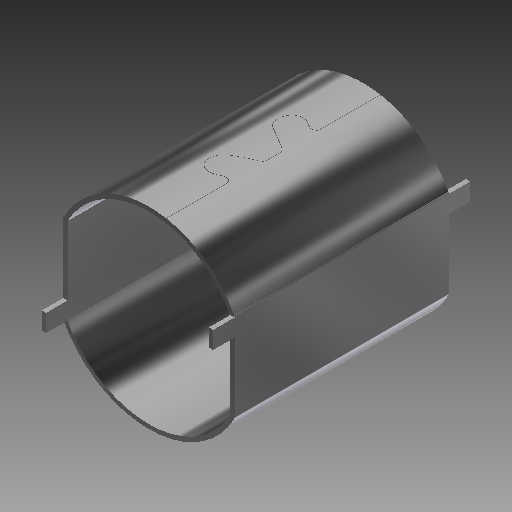
# Autodesk Inventor part: M-001
Saved by Autodesk Inventor 2019 (Build 230136000, 136)
## iProperties
Company: Autodesk Inc.
Created: 2007-10-30
Part Number: M-001
Document SubType Name: Sheet Metal
Designer: Autodesk Inc.
Density: 8 g/cm^3
Mass: 55.2333 g
Surface Area: 142.635 cm^2
Volume: 6.90416 cm^3
Material: Stainless Steel
Description: MOTOR SLEEVE
Sheet Metal Rule: Default
Appearance: Semi-Polished
Component Category: Electrical
Author: Inventor
Autodesk Inventor part; units mm, degrees
ref_plane "YZ Plane" through (0, 0, 0) normal (1, 0, 0) x (0, 1, 0)
ref_plane "XY Plane" through (0, 0, 0) normal (0, 0, 1) x (1, 0, 0)
sketch "Sketch1" plane through (0, 0, 0) normal (0, 0, 1) x (1, 0, 0)
  line L0 (-20, 10.0611) -> (-20, -10.0611)
  line L1 (20, 10.0611) -> (20, -10.0611)
  arc A0 (-19.8831, -10.5315) -> (19.8831, -10.5315) centre (0, 0) ccw
  arc A1 (19.8831, 10.5315) -> (-19.8831, 10.5315) centre (0, 0) ccw
  line L2 (-19, 10.0611) -> (-19, -10.0611)
  arc A2 (-18.9994, -10.0634) -> (19, -10.0623) centre (0, 0) ccw
  line L3 (19, -10.0623) -> (19, 10.0611)
  arc A3 (18.9994, 10.0634) -> (-18.9994, 10.0634) centre (0, 0) ccw
  arc A4 (-18.9994, 10.0634) -> (-19, 10.0611) centre (-18.995, 10.0611) ccw
  arc A5 (19, 10.0611) -> (18.9994, 10.0634) centre (18.995, 10.0611) ccw
  arc A6 (-19, -10.0611) -> (-18.9994, -10.0634) centre (-18.995, -10.0611) ccw
  arc A7 (-19.8831, 10.5315) -> (-20, 10.0611) centre (-18.995, 10.0611) ccw
  arc A8 (-20, -10.0611) -> (-19.8831, -10.5315) centre (-18.995, -10.0611) ccw
  arc A9 (19.8831, -10.5315) -> (20, -10.0611) centre (18.995, -10.0611) ccw
  arc A10 (20, 10.0611) -> (19.8831, 10.5315) centre (18.995, 10.0611) ccw
  dimension "d1" = 40
  dimension "d2" = 20
  dimension "d3" = 22.5
  dimension "d4" = 1
  dimension "d17" = 0.005
  dimension "d19" = 1.005
  dimension "d22" = 22.5
  constraints: 22 point on circle, 14 tangent, 11 centre point, 8 end point, 5 equal radius, 2 parallel, 1 coincident, 1 vertical, 3 other
  measures "d1" distance between parallel lines of L1 L0
  measures "d2" distance from line of L1 point (0, 0)
  measures "d3" radius of A1
  measures "d4" distance between parallel lines of L0 L2
  measures "d17" radius of A4
  measures "d19" radius of A7
  measures "d22" radius of A0
extrude "Extrusion1" add sketch "Sketch1" along normal mid plane 50
ref_plane "Work Plane1" through (0, 22.5, 0) normal (0, 1, 0) x (-1, 0, 0)
sketch "Sketch2" plane through (0, 22.5, 0) normal (0, 1, 0) x (-1, 0, 0)
  line L0 (0, -35) -> (0, 35) projected
  line L1 (-28, 0) -> (28, 0) projected
  line L2 (19.8831, 25) -> (-19.8831, 25) projected
  line L3 (-19.8831, 25) -> (19.8831, 25) projected
  line L4 (-4, 25) -> (-4, 10.8868)
  line L5 (-2.5, 10.0207) -> (-1.5, 10.5981)
  arc A0 (1.5, 5.4019) -> (-1.5, 10.5981) centre (0, 8) ccw
  line L6 (1.5, 5.4019) -> (-3.5, 2.5152)
  line L7 (-4, 1.6491) -> (-4, 0)
  arc A1 (-4, 10.8868) -> (-2.5, 10.0207) centre (-3, 10.8868) ccw
  arc A2 (-3.5, 2.5152) -> (-4, 1.6491) centre (-3, 1.6491) ccw
  line L8 (-4.1, 0) -> (-4.1, 1.6491)
  arc A3 (-3.55, 2.6018) -> (-4.1, 1.6491) centre (-3, 1.6491) ccw
  line L9 (-3.55, 2.6018) -> (1.45, 5.4885)
  arc A4 (1.45, 5.4885) -> (-1.45, 10.5115) centre (0, 8) ccw
  line L10 (-1.45, 10.5115) -> (-2.45, 9.9341)
  arc A5 (-4.1, 10.8868) -> (-2.45, 9.9341) centre (-3, 10.8868) ccw
  line L11 (-4.1, 10.8868) -> (-4.1, 25)
  line L12 (-4, -25) -> (-4, -10.8868)
  line L13 (-2.5, -10.0207) -> (-1.5, -10.5981)
  arc A6 (-1.5, -10.5981) -> (1.5, -5.4019) centre (0, -8) ccw
  line L14 (1.5, -5.4019) -> (-3.5, -2.5152)
  line L15 (-4, -1.6491) -> (-4, 0)
  arc A7 (-2.5, -10.0207) -> (-4, -10.8868) centre (-3, -10.8868) ccw
  arc A8 (-4, -1.6491) -> (-3.5, -2.5152) centre (-3, -1.6491) ccw
  line L16 (-4.1, 0) -> (-4.1, -1.6491)
  arc A9 (-4.1, -1.6491) -> (-3.55, -2.6018) centre (-3, -1.6491) ccw
  line L17 (-3.55, -2.6018) -> (1.45, -5.4885)
  arc A10 (-1.45, -10.5115) -> (1.45, -5.4885) centre (0, -8) ccw
  line L18 (-1.45, -10.5115) -> (-2.45, -9.9341)
  arc A11 (-2.45, -9.9341) -> (-4.1, -10.8868) centre (-3, -10.8868) ccw
  line L19 (-4.1, -10.8868) -> (-4.1, -25)
  line L20 (-4, -25) -> (-4.1, -25)
  line L21 (-4.1, 25) -> (-4, 25)
  line L22 (20, 25) -> (19.8831, 25) projected
  line L23 (19.8831, 25) -> (20, 25) projected
  line L24 (-20, 25) -> (-19.8831, 25) projected
  line L25 (-19.8831, 25) -> (-20, 25) projected
  point P0 (0, 0)
  dimension "d8" = 60
  dimension "d9" = 6
  dimension "d11" = 4
  dimension "d12" = 1
  dimension "d13" = 1
  dimension "d14" = 0.1
  dimension "d21" = 14.1133
  constraints: 36 end point, 24 point on circle, 17 symmetric about line, 12 centre point, 6 tangent, 3 parallel, 3 point on line, 2 collinear, 2 perpendicular, 12 other
  measures "d8" angle of L5 L4
  measures "d9" diameter of A0
  measures "d11" distance between parallel lines of L0 L4
  measures "d12" radius of A1
  measures "d13" radius of A2
  measures "d14" distance between parallel lines of L4 L11
  measures "d21" distance from line of A1.centre L2
extrude "Cut1" cut sketch "Sketch2" against normal blind 3 contours A6 L13 A7 L12 L20 L19 A11 L18 A10 L0 | L0 A10 L17 L14 A6 | L17 A9 L16 L1 L15 A8 L14 L0 | L6 A2 L7 L1 L8 A3 L9 L0 | L0 L9 A4 A0 L6 | A4 L10 A5 L11 L2 L4 A1 L5 A0 L0
sketch "Sketch3" plane through (0, 0, -25) normal (0, 0, -1) x (-1, 0, 0)
  arc A0 (-4.1, 22.1233) -> (-19.8831, 10.5315) centre (0, 0) ccw projected
  line L0 (-20, -10.0611) -> (-20, 10.0611) projected
  line L1 (20, 10.0611) -> (20, -10.0611) projected
  arc A1 (18.9994, -10.0634) -> (19, -10.0611) centre (18.995, -10.0611) ccw projected
  arc A2 (-18.9994, 10.0634) -> (-19, 10.0611) centre (-18.995, 10.0611) ccw projected
  line L2 (18.995, -10.0611) -> (20, -10.0611)
  line L3 (20, -10.0611) -> (20, -6)
  line L4 (20, -6) -> (18.995, -6)
  line L5 (18.995, -6) -> (18.995, -10.0611)
  line L6 (-18.995, 10.0611) -> (-20, 10.0611)
  line L7 (-20, 10.0611) -> (-20, 6)
  line L8 (-20, 6) -> (-18.995, 6)
  line L9 (-18.995, 6) -> (-18.995, 10.0611)
  dimension "d23" = 6
  dimension "d24" = 6
  constraints: 16 end point, 4 parallel, 2 horizontal, 2 perpendicular, 2 point on line
  measures "d23" distance from line of A0.centre L4
  measures "d24" distance from line of A0.centre L8
extrude "Extrusion2" add sketch "Sketch3" along normal blind 5
mirror "Mirror1" about plane through (0, 0, 0) normal (0, 0, 1) of "Extrusion2"
equation "\"d2\" = 0.5 * d1"
equation "\"d22\" = d3"
equation "\"d24\" = d23"
equation "\"BendRadius\" = Thickness"
equation "\"BendReliefWidth\" = Thickness"
equation "\"BendReliefDepth\" = 0.5 * Thickness"
equation "\"CornerReliefSize\" = 4 * Thickness"
equation "\"MinimumRemnant\" = 2 * Thickness"
equation "\"TransitionRadius\" = BendRadius"
equation "\"JacobiRadiusSize\" = Thickness"
equation "\"GapSize\" = Thickness"
equation "\"d27\" = Thickness"
equation "\"Thickness\" = 1"
body "Solid1"
